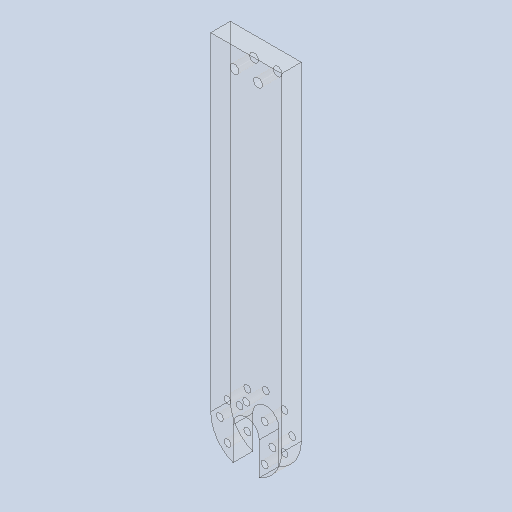
# Autodesk Inventor part: _hand_adt_ver_2_
Saved by Autodesk Inventor 2024.3 (Build 283343000, 343)
## iProperties
Created: 2024-09-07
Part Number: _hand_adt_ver_2_
Material: PMMA 플라스틱
Document SubType Name: Modeling
Designer: gretc
Density: 1.188 g/cm^3
Appearance: 폴리카보네이트 - 선명
Mass: 15.6674 g
Surface Area: 64.5468 cm^2
Volume: 13.188 cm^3
Author: gretc
Autodesk Inventor part; units mm, degrees
ref_plane "YZ Plane" through (0, 0, 0) normal (1, 0, 0) x (0, 1, 0)
ref_plane "XZ Plane" through (0, 0, 0) normal (0, 1, 0) x (-1, 0, 0)
ref_plane "XY Plane" through (0, 0, 0) normal (0, 0, 1) x (1, 0, 0)
sketch "스케치1" plane through (0, 0, 0) normal (0, 0, 1) x (1, 0, 0)
  circle A0 centre (0, 0) radius 10.8 projected
  circle A1 centre (0, 0) radius 6 projected
  circle A2 centre (0, -8) radius 1.05 projected
  circle A3 centre (-5.6569, -5.6569) radius 1.05 projected
  circle A4 centre (-8, 0) radius 1.05 projected
  circle A5 centre (-5.6569, 5.6569) radius 1.05 projected
  circle A6 centre (0, 8) radius 1.05 projected
  circle A7 centre (5.6569, 5.6569) radius 1.05 projected
  circle A8 centre (8, 0) radius 1.05 projected
  circle A9 centre (5.6569, -5.6569) radius 1.05 projected
  circle A10 centre (0, 0) radius 3.6 projected
  circle A11 centre (0, 0) radius 3.6 projected
  circle A12 centre (0, 0) radius 4
  line L0 (-4, 0) -> (4, 0)
  line L1 (4, 0) -> (4, -13.3653)
  line L2 (4, -13.3653) -> (-4, -13.3653)
  line L3 (-4, -13.3653) -> (-4, 0)
  line L4 (-10.8, 0) -> (10.8, 0)
  line L5 (10.8, 0) -> (10.8, 100)
  line L6 (10.8, 100) -> (-10.8, 100)
  line L7 (-10.8, 100) -> (-10.8, 0)
  line L8 (10.8, 100) -> (10.8, 94)
  line L9 (10.8, 94) -> (3.6, 94)
  line L10 (3.6, 94) -> (-3.6, 94)
  line L11 (-3.6, 94) -> (-10.8, 94)
  circle A13 centre (-3.6, 94) radius 1.35
  circle A14 centre (3.6, 94) radius 1.35
  point P0 (0, 0)
  point P1 (-3.6, 0)
  point P2 (3.6, 0)
  point P3 (-4, -10.0319)
  point P4 (4, -10.0319)
  dimension "d0" = 8
  dimension "d1" = 100
  dimension "d2" = 21.6
  dimension "d3" = 6
  dimension "d4" = 7.2
  dimension "d5" = 7.2
  dimension "d6" = 2.7
  dimension "d7" = 2.7
  constraints: 24 end point, 6 point on circle, 4 parallel, 4 point on line, 3 centre point, 3 coincident, 3 perpendicular, 2 horizontal
  measures "d0" diameter of A12
  measures "d1" distance of L5.end L4.end
  measures "d2" distance between parallel lines of L5 L7
  measures "d3" distance of L5.end L8.end
  measures "d4" distance of L8.end L9.end
  measures "d5" distance of L9.end L10.end
  measures "d6" diameter of A13
  measures "d7" diameter of A14
extrude "돌출1" add sketch "스케치1" along normal blind 6 contours L4 A8 A1 A4 A0 | A0 L1 A1 L4 A8 | A0 L7 L11 A13 L10 A14 L9 L5 | L4 A4 A1 L3 A0 | L9 A14 L10 A13 L11 L7 L6 L5 | L1 L4 A1 | A1 L4 L3 | L4 A12 A1
